Autodesk Fusion 360 part; units mm, degrees
note: some values were not read from the file. Chosen so that the rebuilt part matches the saved one: which bodies a step acts on.
(part 2 of 4)
  arc A344 (288.775, -83.4875) -> (288.275, -83.9875) centre (288.775, -83.9875) ccw
  arc A345 (302.275, -83.9875) -> (301.775, -83.4875) centre (301.775, -83.9875) ccw
  arc A346 (288.275, -96.9875) -> (288.775, -97.4875) centre (288.775, -96.9875) ccw
  arc A347 (301.775, -97.4875) -> (302.275, -96.9875) centre (301.775, -96.9875) ccw
  line L378 (5.4062, -102.5375) -> (18.4063, -102.5375)
  line L379 (5.4062, -116.5375) -> (18.4063, -116.5375)
  line L380 (4.9062, -103.0375) -> (4.9062, -116.0375)
  line L381 (18.9062, -103.0375) -> (18.9062, -116.0375)
  arc A348 (5.4062, -102.5375) -> (4.9062, -103.0375) centre (5.4062, -103.0375) ccw
  arc A349 (18.9062, -103.0375) -> (18.4062, -102.5375) centre (18.4062, -103.0375) ccw
  arc A350 (4.9062, -116.0375) -> (5.4062, -116.5375) centre (5.4062, -116.0375) ccw
  arc A351 (18.4062, -116.5375) -> (18.9063, -116.0375) centre (18.4062, -116.0375) ccw
  line L382 (29.2188, -102.5375) -> (42.2188, -102.5375)
  line L383 (29.2188, -116.5375) -> (42.2188, -116.5375)
  line L384 (28.7188, -103.0375) -> (28.7188, -116.0375)
  line L385 (42.7188, -103.0375) -> (42.7188, -116.0375)
  arc A352 (29.2188, -102.5375) -> (28.7187, -103.0375) centre (29.2188, -103.0375) ccw
  arc A353 (42.7188, -103.0375) -> (42.2188, -102.5375) centre (42.2188, -103.0375) ccw
  arc A354 (28.7188, -116.0375) -> (29.2188, -116.5375) centre (29.2188, -116.0375) ccw
  arc A355 (42.2188, -116.5375) -> (42.7188, -116.0375) centre (42.2188, -116.0375) ccw
  line L386 (55.4125, -102.5375) -> (68.4125, -102.5375)
  line L387 (55.4125, -116.5375) -> (68.4125, -116.5375)
  line L388 (54.9125, -103.0375) -> (54.9125, -116.0375)
  line L389 (68.9125, -103.0375) -> (68.9125, -116.0375)
  arc A356 (55.4125, -102.5375) -> (54.9125, -103.0375) centre (55.4125, -103.0375) ccw
  arc A357 (68.9125, -103.0375) -> (68.4125, -102.5375) centre (68.4125, -103.0375) ccw
  arc A358 (54.9125, -116.0375) -> (55.4125, -116.5375) centre (55.4125, -116.0375) ccw
  arc A359 (68.4125, -116.5375) -> (68.9125, -116.0375) centre (68.4125, -116.0375) ccw
  line L390 (129.2312, -102.5375) -> (142.2312, -102.5375)
  line L391 (129.2312, -116.5375) -> (142.2312, -116.5375)
  line L392 (128.7312, -103.0375) -> (128.7312, -116.0375)
  line L393 (142.7312, -103.0375) -> (142.7312, -116.0375)
  arc A360 (129.2312, -102.5375) -> (128.7312, -103.0375) centre (129.2312, -103.0375) ccw
  arc A361 (142.7312, -103.0375) -> (142.2312, -102.5375) centre (142.2312, -103.0375) ccw
  arc A362 (128.7312, -116.0375) -> (129.2312, -116.5375) centre (129.2312, -116.0375) ccw
  arc A363 (142.2312, -116.5375) -> (142.7312, -116.0375) centre (142.2312, -116.0375) ccw
  line L394 (82.9039, -103.8479) -> (88.5587, -103.8479)
  line L395 (89.0587, -104.3479) -> (89.0587, -106.7375)
  line L396 (89.5587, -107.2375) -> (135.7312, -107.2375)
  line L397 (135.7312, -111.8375) -> (89.5587, -111.8375)
  line L398 (89.0587, -112.3375) -> (89.0587, -115.6415)
  line L399 (88.5587, -116.1415) -> (87.7553, -116.1415)
  line L400 (87.2553, -116.6415) -> (87.2553, -116.8099)
  line L401 (86.7553, -117.3099) -> (84.7073, -117.3099)
  line L402 (84.2073, -116.8099) -> (84.2073, -116.6415)
  line L403 (83.7073, -116.1415) -> (82.9039, -116.1415)
  line L404 (82.4039, -115.6415) -> (82.4039, -110.5455)
  line L405 (81.9039, -110.0455) -> (81.5403, -110.0455)
  line L406 (81.5403, -110.0455) -> (81.5403, -107.7515)
  line L407 (82.0403, -107.2515) -> (82.4039, -107.2515)
  line L408 (82.4039, -107.2515) -> (82.4039, -104.3479)
  arc A364 (89.0587, -104.3479) -> (88.5587, -103.8479) centre (88.5587, -104.3479) ccw
  arc A365 (89.0587, -106.7375) -> (89.5587, -107.2375) centre (89.5587, -106.7375) ccw
  arc A366 (89.5587, -111.8375) -> (89.0587, -112.3375) centre (89.5587, -112.3375) ccw
  arc A367 (88.5587, -116.1415) -> (89.0587, -115.6415) centre (88.5587, -115.6415) ccw
  arc A368 (87.7553, -116.1415) -> (87.2553, -116.6415) centre (87.7553, -116.6415) ccw
  arc A369 (86.7553, -117.3099) -> (87.2552, -116.8099) centre (86.7553, -116.8099) ccw
  arc A370 (84.2073, -116.8099) -> (84.7073, -117.3099) centre (84.7073, -116.8099) ccw
  arc A371 (84.2073, -116.6415) -> (83.7073, -116.1415) centre (83.7073, -116.6415) ccw
  arc A372 (82.4039, -115.6415) -> (82.9039, -116.1415) centre (82.9039, -115.6415) ccw
  arc A373 (82.4039, -110.5455) -> (81.9039, -110.0455) centre (81.9039, -110.5455) ccw
  arc A374 (82.0403, -107.2515) -> (81.5402, -107.7515) centre (82.0403, -107.7515) ccw
  arc A375 (82.9039, -103.8479) -> (82.4039, -104.3479) centre (82.9039, -104.3479) ccw
  line L409 (188.5587, -103.8479) -> (182.9038, -103.8479)
  line L410 (182.4039, -104.3479) -> (182.4039, -106.7375)
  line L411 (181.9039, -107.2375) -> (135.7312, -107.2375)
  line L412 (135.7312, -111.8375) -> (181.9039, -111.8375)
  line L413 (182.4039, -112.3375) -> (182.4039, -115.6415)
  line L414 (182.9039, -116.1415) -> (183.7072, -116.1415)
  line L415 (184.2073, -116.6415) -> (184.2073, -116.8099)
  line L416 (184.7072, -117.3099) -> (186.7553, -117.3099)
  line L417 (187.2553, -116.8099) -> (187.2553, -116.6415)
  line L418 (187.7552, -116.1415) -> (188.5587, -116.1415)
  line L419 (189.0587, -115.6415) -> (189.0587, -110.5455)
  line L420 (189.5587, -110.0455) -> (189.9223, -110.0455)
  line L421 (189.9223, -110.0455) -> (189.9223, -107.7515)
  line L422 (189.4223, -107.2515) -> (189.0587, -107.2515)
  line L423 (189.0587, -107.2515) -> (189.0587, -104.3479)
  arc A376 (182.9039, -103.8479) -> (182.4039, -104.3479) centre (182.9039, -104.3479) ccw
  arc A377 (181.9039, -107.2375) -> (182.4039, -106.7375) centre (181.9039, -106.7375) ccw
  arc A378 (182.4039, -112.3375) -> (181.9039, -111.8375) centre (181.9039, -112.3375) ccw
  arc A379 (182.4039, -115.6415) -> (182.9039, -116.1415) centre (182.9039, -115.6415) ccw
  arc A380 (184.2072, -116.6415) -> (183.7072, -116.1415) centre (183.7072, -116.6415) ccw
  arc A381 (184.2073, -116.8099) -> (184.7072, -117.3099) centre (184.7072, -116.8099) ccw
  arc A382 (186.7552, -117.3099) -> (187.2552, -116.8099) centre (186.7552, -116.8099) ccw
  arc A383 (187.7552, -116.1415) -> (187.2552, -116.6415) centre (187.7552, -116.6415) ccw
  arc A384 (188.5587, -116.1415) -> (189.0587, -115.6415) centre (188.5587, -115.6415) ccw
  arc A385 (189.5587, -110.0455) -> (189.0587, -110.5455) centre (189.5587, -110.5455) ccw
  arc A386 (189.9223, -107.7515) -> (189.4223, -107.2515) centre (189.4223, -107.7515) ccw
  arc A387 (189.0587, -104.3479) -> (188.5587, -103.8479) centre (188.5587, -104.3479) ccw
  line L424 (203.05, -102.5375) -> (216.05, -102.5375)
  line L425 (203.05, -116.5375) -> (216.05, -116.5375)
  line L426 (202.55, -103.0375) -> (202.55, -116.0375)
  line L427 (216.55, -103.0375) -> (216.55, -116.0375)
  arc A388 (203.05, -102.5375) -> (202.55, -103.0375) centre (203.05, -103.0375) ccw
  arc A389 (216.55, -103.0375) -> (216.05, -102.5375) centre (216.05, -103.0375) ccw
  arc A390 (202.55, -116.0375) -> (203.05, -116.5375) centre (203.05, -116.0375) ccw
  arc A391 (216.05, -116.5375) -> (216.55, -116.0375) centre (216.05, -116.0375) ccw
  line L428 (229.2438, -102.5375) -> (242.2438, -102.5375)
  line L429 (229.2438, -116.5375) -> (242.2438, -116.5375)
  line L430 (228.7438, -103.0375) -> (228.7438, -116.0375)
  line L431 (242.7438, -103.0375) -> (242.7438, -116.0375)
  arc A392 (229.2438, -102.5375) -> (228.7438, -103.0375) centre (229.2438, -103.0375) ccw
  arc A393 (242.7438, -103.0375) -> (242.2438, -102.5375) centre (242.2438, -103.0375) ccw
  arc A394 (228.7438, -116.0375) -> (229.2438, -116.5375) centre (229.2438, -116.0375) ccw
  arc A395 (242.2438, -116.5375) -> (242.7438, -116.0375) centre (242.2438, -116.0375) ccw
  line L432 (250.675, -102.5375) -> (263.675, -102.5375)
  line L433 (250.675, -116.5375) -> (263.675, -116.5375)
  line L434 (250.175, -103.0375) -> (250.175, -116.0375)
  line L435 (264.175, -103.0375) -> (264.175, -116.0375)
  arc A396 (250.675, -102.5375) -> (250.175, -103.0375) centre (250.675, -103.0375) ccw
  arc A397 (264.175, -103.0375) -> (263.675, -102.5375) centre (263.675, -103.0375) ccw
  arc A398 (250.175, -116.0375) -> (250.675, -116.5375) centre (250.675, -116.0375) ccw
  arc A399 (263.675, -116.5375) -> (264.175, -116.0375) centre (263.675, -116.0375) ccw
  line L436 (269.725, -102.5375) -> (282.725, -102.5375)
  line L437 (269.725, -116.5375) -> (282.725, -116.5375)
  line L438 (269.225, -103.0375) -> (269.225, -116.0375)
  line L439 (283.225, -103.0375) -> (283.225, -116.0375)
  arc A400 (269.725, -102.5375) -> (269.225, -103.0375) centre (269.725, -103.0375) ccw
  arc A401 (283.225, -103.0375) -> (282.725, -102.5375) centre (282.725, -103.0375) ccw
  arc A402 (269.225, -116.0375) -> (269.725, -116.5375) centre (269.725, -116.0375) ccw
  arc A403 (282.725, -116.5375) -> (283.225, -116.0375) centre (282.725, -116.0375) ccw
  line L440 (288.775, -102.5375) -> (301.775, -102.5375)
  line L441 (288.775, -116.5375) -> (301.775, -116.5375)
  line L442 (288.275, -103.0375) -> (288.275, -116.0375)
  line L443 (302.275, -103.0375) -> (302.275, -116.0375)
  arc A404 (288.775, -102.5375) -> (288.275, -103.0375) centre (288.775, -103.0375) ccw
  arc A405 (302.275, -103.0375) -> (301.775, -102.5375) centre (301.775, -103.0375) ccw
  arc A406 (288.275, -116.0375) -> (288.775, -116.5375) centre (288.775, -116.0375) ccw
  arc A407 (301.775, -116.5375) -> (302.275, -116.0375) centre (301.775, -116.0375) ccw
  line L444 (0, -120.1996) -> (304.8, -120.1996)
  line L445 (0, 0) -> (304.8, 0)
  line L446 (0, -120.1996) -> (0, 0)
  line L447 (304.8, -120.1996) -> (304.8, 0)
  circle A408 centre (295.243, -9.275) radius 3.25
  line L448 (300.493, -15.275) -> (289.993, -15.275)
  line L449 (289.243, -14.525) -> (289.243, -4.025)
  line L450 (289.993, -3.275) -> (300.493, -3.275)
  line L451 (301.243, -4.025) -> (301.243, -14.525)
  line L452 (301.243, -15.275) -> (289.243, -3.275) construction
  line L453 (289.243, -15.275) -> (301.243, -3.275) construction
  arc A409 (301.243, -4.025) -> (300.493, -3.275) centre (300.493, -4.025) ccw
  arc A410 (300.493, -15.275) -> (301.243, -14.525) centre (300.493, -14.525) ccw
  arc A411 (289.243, -14.525) -> (289.993, -15.275) centre (289.993, -14.525) ccw
  arc A412 (289.993, -3.275) -> (289.243, -4.025) centre (289.993, -4.025) ccw
  line L454 (-4, 10) -> (308.8, 10)
  line L455 (308.8, 10) -> (308.8, -130.1996)
  line L456 (308.8, -130.1996) -> (-4, -130.1996)
  line L457 (-4, -130.1996) -> (-4, 10)
  line L458 (273.8, 10) -> (202.4, 10)
  line L459 (202.4, 10) -> (202.4, 3)
  line L460 (202.4, 3) -> (273.8, 3)
  line L461 (273.8, 3) -> (273.8, 10)
  line L462 (31, 10) -> (102.4, 10)
  line L463 (102.4, 10) -> (102.4, 3)
  line L464 (102.4, 3) -> (31, 3)
  line L465 (31, 3) -> (31, 10)
  line L466 (152.4, 0) -> (152.4, 19)
  line L467 (31, -130.1996) -> (102.4, -130.1996)
  line L468 (102.4, -130.1996) -> (102.4, -123.1996)
  line L469 (102.4, -123.1996) -> (31, -123.1996)
  line L470 (31, -123.1996) -> (31, -130.1996)
  line L471 (273.8, -130.1996) -> (202.4, -130.1996)
  line L472 (202.4, -130.1996) -> (202.4, -123.1996)
  line L473 (202.4, -123.1996) -> (273.8, -123.1996)
  line L474 (273.8, -123.1996) -> (273.8, -130.1996)
  line L475 (152.4, -120.1996) -> (152.4, -154.1242)
  point P0 (295.243, -9.275)
  dimension "d1" = 6.5
  dimension "d6" = 12
  dimension "d7" = 0.75
  dimension "d9" = 12
  dimension "d10" = 7
  dimension "d11" = 14
  dimension "d12" = 6.7539
  dimension "d13" = 10
  dimension "d14" = 4
  dimension "d15" = 10
  dimension "d16" = 4
  dimension "d19" = 2.525
  dimension "d20" = 2.525
  dimension "d21" = 35
  dimension "d22" = 7
  dimension "d23" = 100
  dimension "d24" = 35
  dimension "d25" = 7
  dimension "d26" = 50
  dimension "d27" = 35
  dimension "d28" = 35
  dimension "d29" = 100
  dimension "d30" = 50
  dimension "d31" = 7
  dimension "d32" = 7
  dimension "d37" = 71.4
  constraint horizontal L448
  constraint perpendicular L448 L449
  constraint parallel L448 L450
  constraint parallel L449 L451
  constraint coincident L452 P0
  constraint coincident L453 P0
  constraint coincident P0 A408.centre
  constraint coincident L453.end L451
  constraint coincident L453.end L450
  constraint tangent L451 A409
  constraint tangent L450 A409
  constraint coincident L452.start L448
  constraint coincident L452.start L451
  constraint tangent L448 A410
  constraint tangent L451 A410
  constraint equal A409 A410
  constraint coincident L453.start L449
  constraint coincident L453.start L448
  constraint tangent L449 A411
  constraint tangent L448 A411
  constraint equal A409 A411
  constraint coincident L452.end L449
  constraint coincident L452.end L450
  constraint tangent L449 A412
  constraint tangent L450 A412
  constraint equal A409 A412
  constraint horizontal L454
  constraint vertical L455
  constraint horizontal L456
  constraint vertical L457
  constraint horizontal L458
  constraint vertical L459
  constraint horizontal L460
  constraint vertical L461
  constraint coincident L454 L458.start
  constraint horizontal L462
  constraint vertical L463
  constraint horizontal L464
  constraint vertical L465
  constraint coincident L454 L462.start
  constraint midpoint L445 L466.start
  constraint perpendicular L454 L466
  constraint horizontal L467
  constraint vertical L468
  constraint horizontal L469
  constraint vertical L470
  constraint coincident L456 L467.start
  constraint horizontal L471
  constraint vertical L472
  constraint horizontal L473
  constraint vertical L474
  constraint coincident L456 L471.start
  constraint equal L460 L473
  constraint equal L464 L469
  constraint midpoint L444 L475.start
  constraint perpendicular L456 L475
  measures "d1" diameter of A408
  measures "d6" distance of L453.start L452.end
  measures "d7" radius of A409
  measures "d9" distance of L451.start L449.end
  measures "d10" distance of L54 P0
  measures "d11" distance of L50 L51
  measures "d12" distance of L52 P0
  measures "d13" distance of L444 L456
  measures "d14" distance of L447 L455
  measures "d15" distance of L445 L454
  measures "d16" distance of L446 L457
  measures "d19" distance of L2 L446
  measures "d20" distance of L145 L447
  measures "d21" distance of L454.start L462.start
  measures "d22" distance of L454 L464
  measures "d23" distance of L459 L463
  measures "d24" distance of L455 L461
  measures "d25" distance of L454 L460
  measures "d26" distance of L463 L466
  measures "d27" distance of L455.end L471.start
  measures "d28" distance of L456.end L467.start
  measures "d29" distance of L467.end L471.end
  measures "d30" distance of L467.end L475
  measures "d31" distance of L467 L469
  measures "d32" distance of L471 L473
  measures "d37" distance of L463 L465
extrude "Extrude1" add sketch "Plate May 11 2026" along normal blind 3 contours L444 L445 L446 L447 | L444 L445 L446 L454 L456 L457 L463 L464 L465 L466 L468 L469 L470 L475 | L444 L445 L447 L454 L455 L456 L459 L460 L461 L466 L472 L473 L474 L475 makes body 1
fillet "Fillet1" radius 5 4 edges at (308.8, -130.1996, 1.5) (-4, -130.1996, 1.5) (308.8, 10, 1.5) (-4, 10, 1.5) on bodies 1
fillet "Fillet2" radius 5 4 edges at (31, 10, 1.5) (202.4, 10, 1.5) (102.4, 10, 1.5) (273.8, 10, 1.5) on bodies 1
fillet "Fillet3" radius 5 4 edges at (273.8, -130.1996, 1.5) (202.4, -130.1996, 1.5) (102.4, -130.1996, 1.5) (31, -130.1996, 1.5) on bodies 1
ref_plane "WorkPlane1" through (156.4, 0, 0) normal (1, 0, 0) x (0, 1, 0)
sketch "Sketch2" plane through (0, 0, 0) normal (0, 0, -1) x (1, 0, 0)
  arc A0 (216.8375, 83.9875) -> (217.3375, 83.4875) centre (217.3375, 83.9875) ccw
  line L0 (216.8375, 83.9875) -> (216.8375, 96.9875)
  arc A1 (217.3375, 97.4875) -> (216.8375, 96.9875) centre (217.3375, 96.9875) ccw
  line L1 (217.3375, 97.4875) -> (230.3375, 97.4875)
  arc A2 (230.8375, 96.9875) -> (230.3375, 97.4875) centre (230.3375, 96.9875) ccw
  line L2 (230.8375, 96.9875) -> (230.8375, 83.9875)
  arc A3 (230.3375, 83.4875) -> (230.8375, 83.9875) centre (230.3375, 83.9875) ccw
  line L3 (230.3375, 83.4875) -> (217.3375, 83.4875)
  arc A4 (50.15, 45.8875) -> (50.65, 45.3875) centre (50.65, 45.8875) ccw
  line L4 (50.15, 45.8875) -> (50.15, 58.8875)
  arc A5 (50.65, 59.3875) -> (50.15, 58.8875) centre (50.65, 58.8875) ccw
  line L5 (50.65, 59.3875) -> (63.65, 59.3875)
  arc A6 (64.15, 58.8875) -> (63.65, 59.3875) centre (63.65, 58.8875) ccw
  line L6 (64.15, 58.8875) -> (64.15, 45.8875)
  arc A7 (63.65, 45.3875) -> (64.15, 45.8875) centre (63.65, 45.8875) ccw
  line L7 (63.65, 45.3875) -> (50.65, 45.3875)
  arc A8 (288.275, 26.8375) -> (288.775, 26.3375) centre (288.775, 26.8375) ccw
  line L8 (288.275, 26.8375) -> (288.275, 39.8375)
  arc A9 (288.775, 40.3375) -> (288.275, 39.8375) centre (288.775, 39.8375) ccw
  line L9 (288.775, 40.3375) -> (301.775, 40.3375)
  arc A10 (302.275, 39.8375) -> (301.775, 40.3375) centre (301.775, 39.8375) ccw
  line L10 (302.275, 39.8375) -> (302.275, 26.8375)
  arc A11 (301.775, 26.3375) -> (302.275, 26.8375) centre (301.775, 26.8375) ccw
  line L11 (301.775, 26.3375) -> (288.775, 26.3375)
  arc A12 (169.2125, 64.9375) -> (169.7125, 64.4375) centre (169.7125, 64.9375) ccw
  line L12 (169.2125, 64.9375) -> (169.2125, 77.9375)
  arc A13 (169.7125, 78.4375) -> (169.2125, 77.9375) centre (169.7125, 77.9375) ccw
  line L13 (169.7125, 78.4375) -> (182.7125, 78.4375)
  arc A14 (183.2125, 77.9375) -> (182.7125, 78.4375) centre (182.7125, 77.9375) ccw
  line L14 (183.2125, 77.9375) -> (183.2125, 64.9375)
  arc A15 (182.7125, 64.4375) -> (183.2125, 64.9375) centre (182.7125, 64.9375) ccw
  line L15 (182.7125, 64.4375) -> (169.7125, 64.4375)
  arc A16 (31.1, 45.8875) -> (31.6, 45.3875) centre (31.6, 45.8875) ccw
  line L16 (31.1, 45.8875) -> (31.1, 58.8875)
  arc A17 (31.6, 59.3875) -> (31.1, 58.8875) centre (31.6, 58.8875) ccw
  line L17 (31.6, 59.3875) -> (44.6, 59.3875)
  arc A18 (45.1, 58.8875) -> (44.6, 59.3875) centre (44.6, 58.8875) ccw
  line L18 (45.1, 58.8875) -> (45.1, 45.8875)
  arc A19 (44.6, 45.3875) -> (45.1, 45.8875) centre (44.6, 45.8875) ccw
  line L19 (44.6, 45.3875) -> (31.6, 45.3875)
  arc A20 (7.2875, 45.8875) -> (7.7875, 45.3875) centre (7.7875, 45.8875) ccw
  line L20 (7.2875, 45.8875) -> (7.2875, 58.8875)
  arc A21 (7.7875, 59.3875) -> (7.2875, 58.8875) centre (7.7875, 58.8875) ccw
  line L21 (7.7875, 59.3875) -> (20.7875, 59.3875)
  arc A22 (21.2875, 58.8875) -> (20.7875, 59.3875) centre (20.7875, 58.8875) ccw
  line L22 (21.2875, 58.8875) -> (21.2875, 45.8875)
  arc A23 (20.7875, 45.3875) -> (21.2875, 45.8875) centre (20.7875, 45.8875) ccw
  line L23 (20.7875, 45.3875) -> (7.7875, 45.3875)
  arc A24 (54.9125, 103.0375) -> (55.4125, 102.5375) centre (55.4125, 103.0375) ccw
  line L24 (54.9125, 103.0375) -> (54.9125, 116.0375)
  arc A25 (55.4125, 116.5375) -> (54.9125, 116.0375) centre (55.4125, 116.0375) ccw
  line L25 (55.4125, 116.5375) -> (68.4125, 116.5375)
  arc A26 (68.9125, 116.0375) -> (68.4125, 116.5375) centre (68.4125, 116.0375) ccw
  line L26 (68.9125, 116.0375) -> (68.9125, 103.0375)
  arc A27 (68.4125, 102.5375) -> (68.9125, 103.0375) centre (68.4125, 103.0375) ccw
  line L27 (68.4125, 102.5375) -> (55.4125, 102.5375)
  arc A28 (54.9125, 3.025) -> (55.4125, 2.525) centre (55.4125, 3.025) ccw
  line L28 (54.9125, 3.025) -> (54.9125, 16.025)
  arc A29 (55.4125, 16.525) -> (54.9125, 16.025) centre (55.4125, 16.025) ccw
  line L29 (55.4125, 16.525) -> (68.4125, 16.525)
  arc A30 (68.9125, 16.025) -> (68.4125, 16.525) centre (68.4125, 16.025) ccw
  line L30 (68.9125, 16.025) -> (68.9125, 3.025)
  arc A31 (68.4125, 2.525) -> (68.9125, 3.025) centre (68.4125, 3.025) ccw
  line L31 (68.4125, 2.525) -> (55.4125, 2.525)
  arc A32 (288.275, 64.9375) -> (288.775, 64.4375) centre (288.775, 64.9375) ccw
  line L32 (288.275, 64.9375) -> (288.275, 77.9375)
  arc A33 (288.775, 78.4375) -> (288.275, 77.9375) centre (288.775, 77.9375) ccw
  line L33 (288.775, 78.4375) -> (301.775, 78.4375)
  arc A34 (302.275, 77.9375) -> (301.775, 78.4375) centre (301.775, 77.9375) ccw
  line L34 (302.275, 77.9375) -> (302.275, 64.9375)
  arc A35 (301.775, 64.4375) -> (302.275, 64.9375) centre (301.775, 64.9375) ccw
  line L35 (301.775, 64.4375) -> (288.775, 64.4375)
  arc A36 (269.225, 83.9875) -> (269.725, 83.4875) centre (269.725, 83.9875) ccw
  line L36 (269.225, 83.9875) -> (269.225, 96.9875)
  arc A37 (269.725, 97.4875) -> (269.225, 96.9875) centre (269.725, 96.9875) ccw
  line L37 (269.725, 97.4875) -> (282.725, 97.4875)
  arc A38 (283.225, 96.9875) -> (282.725, 97.4875) centre (282.725, 96.9875) ccw
  line L38 (283.225, 96.9875) -> (283.225, 83.9875)
  arc A39 (282.725, 83.4875) -> (283.225, 83.9875) centre (282.725, 83.9875) ccw
  line L39 (282.725, 83.4875) -> (269.725, 83.4875)
  arc A40 (73.9625, 3.025) -> (74.4625, 2.525) centre (74.4625, 3.025) ccw
  line L40 (73.9625, 3.025) -> (73.9625, 16.025)
  arc A41 (74.4625, 16.525) -> (73.9625, 16.025) centre (74.4625, 16.025) ccw
  line L41 (74.4625, 16.525) -> (87.4625, 16.525)
  arc A42 (87.9625, 16.025) -> (87.4625, 16.525) centre (87.4625, 16.025) ccw
  line L42 (87.9625, 16.025) -> (87.9625, 3.025)
  arc A43 (87.4625, 2.525) -> (87.9625, 3.025) centre (87.4625, 3.025) ccw
  line L43 (87.4625, 2.525) -> (74.4625, 2.525)
  arc A44 (121.5875, 3.025) -> (122.0875, 2.525) centre (122.0875, 3.025) ccw
  line L44 (121.5875, 3.025) -> (121.5875, 16.025)
  arc A45 (122.0875, 16.525) -> (121.5875, 16.025) centre (122.0875, 16.025) ccw
  line L45 (122.0875, 16.525) -> (135.0875, 16.525)
  arc A46 (135.5875, 16.025) -> (135.0875, 16.525) centre (135.0875, 16.025) ccw
  line L46 (135.5875, 16.025) -> (135.5875, 3.025)
  arc A47 (135.0875, 2.525) -> (135.5875, 3.025) centre (135.0875, 3.025) ccw
  line L47 (135.0875, 2.525) -> (122.0875, 2.525)
  arc A48 (45.3875, 83.9875) -> (45.8875, 83.4875) centre (45.8875, 83.9875) ccw
  line L48 (45.3875, 83.9875) -> (45.3875, 96.9875)
  arc A49 (45.8875, 97.4875) -> (45.3875, 96.9875) centre (45.8875, 96.9875) ccw
  line L49 (45.8875, 97.4875) -> (58.8875, 97.4875)
  arc A50 (59.3875, 96.9875) -> (58.8875, 97.4875) centre (58.8875, 96.9875) ccw
  line L50 (59.3875, 96.9875) -> (59.3875, 83.9875)
  arc A51 (58.8875, 83.4875) -> (59.3875, 83.9875) centre (58.8875, 83.9875) ccw
  line L51 (58.8875, 83.4875) -> (45.8875, 83.4875)
  arc A52 (154.925, 26.8375) -> (155.425, 26.3375) centre (155.425, 26.8375) ccw
  line L52 (154.925, 26.8375) -> (154.925, 39.8375)
  arc A53 (155.425, 40.3375) -> (154.925, 39.8375) centre (155.425, 39.8375) ccw
  line L53 (155.425, 40.3375) -> (168.425, 40.3375)
  arc A54 (168.925, 39.8375) -> (168.425, 40.3375) centre (168.425, 39.8375) ccw
  line L54 (168.925, 39.8375) -> (168.925, 26.8375)
  arc A55 (168.425, 26.3375) -> (168.925, 26.8375) centre (168.425, 26.8375) ccw
  line L55 (168.425, 26.3375) -> (155.425, 26.3375)
  arc A56 (35.8625, 64.9375) -> (36.3625, 64.4375) centre (36.3625, 64.9375) ccw
  line L56 (35.8625, 64.9375) -> (35.8625, 77.9375)
  arc A57 (36.3625, 78.4375) -> (35.8625, 77.9375) centre (36.3625, 77.9375) ccw
  line L57 (36.3625, 78.4375) -> (49.3625, 78.4375)
  arc A58 (49.8625, 77.9375) -> (49.3625, 78.4375) centre (49.3625, 77.9375) ccw
  line L58 (49.8625, 77.9375) -> (49.8625, 64.9375)
  arc A59 (49.3625, 64.4375) -> (49.8625, 64.9375) centre (49.3625, 64.9375) ccw
  line L59 (49.3625, 64.4375) -> (36.3625, 64.4375)
  arc A60 (264.4625, 45.8875) -> (264.9625, 45.3875) centre (264.9625, 45.8875) ccw
  line L60 (264.4625, 45.8875) -> (264.4625, 58.8875)
  arc A61 (264.9625, 59.3875) -> (264.4625, 58.8875) centre (264.9625, 58.8875) ccw
  line L61 (264.9625, 59.3875) -> (277.9625, 59.3875)
  arc A62 (278.4625, 58.8875) -> (277.9625, 59.3875) centre (277.9625, 58.8875) ccw
  line L62 (278.4625, 58.8875) -> (278.4625, 45.8875)
  arc A63 (277.9625, 45.3875) -> (278.4625, 45.8875) centre (277.9625, 45.8875) ccw
  line L63 (277.9625, 45.3875) -> (264.9625, 45.3875)
  arc A64 (288.275, 45.8875) -> (288.775, 45.3875) centre (288.775, 45.8875) ccw
  line L64 (288.275, 45.8875) -> (288.275, 58.8875)
  arc A65 (288.775, 59.3875) -> (288.275, 58.8875) centre (288.775, 58.8875) ccw
  line L65 (288.775, 59.3875) -> (301.775, 59.3875)
  arc A66 (302.275, 58.8875) -> (301.775, 59.3875) centre (301.775, 58.8875) ccw
  line L66 (302.275, 58.8875) -> (302.275, 45.8875)
  arc A67 (301.775, 45.3875) -> (302.275, 45.8875) centre (301.775, 45.8875) ccw
  line L67 (301.775, 45.3875) -> (288.775, 45.3875)
  arc A68 (226.3625, 64.9375) -> (226.8625, 64.4375) centre (226.8625, 64.9375) ccw
  line L68 (226.3625, 64.9375) -> (226.3625, 77.9375)
  arc A69 (226.8625, 78.4375) -> (226.3625, 77.9375) centre (226.8625, 77.9375) ccw
  line L69 (226.8625, 78.4375) -> (239.8625, 78.4375)
  arc A70 (240.3625, 77.9375) -> (239.8625, 78.4375) centre (239.8625, 77.9375) ccw
  line L70 (240.3625, 77.9375) -> (240.3625, 64.9375)
  arc A71 (239.8625, 64.4375) -> (240.3625, 64.9375) centre (239.8625, 64.9375) ccw
  line L71 (239.8625, 64.4375) -> (226.8625, 64.4375)
  arc A72 (221.6, 45.8875) -> (222.1, 45.3875) centre (222.1, 45.8875) ccw
  line L72 (221.6, 45.8875) -> (221.6, 58.8875)
  arc A73 (222.1, 59.3875) -> (221.6, 58.8875) centre (222.1, 58.8875) ccw
  line L73 (222.1, 59.3875) -> (235.1, 59.3875)
  arc A74 (235.6, 58.8875) -> (235.1, 59.3875) centre (235.1, 58.8875) ccw
  line L74 (235.6, 58.8875) -> (235.6, 45.8875)
  arc A75 (235.1, 45.3875) -> (235.6, 45.8875) centre (235.1, 45.8875) ccw
  line L75 (235.1, 45.3875) -> (222.1, 45.3875)
  arc A76 (107.3, 45.8875) -> (107.8, 45.3875) centre (107.8, 45.8875) ccw
  line L76 (107.3, 45.8875) -> (107.3, 58.8875)
  arc A77 (107.8, 59.3875) -> (107.3, 58.8875) centre (107.8, 58.8875) ccw
  line L77 (107.8, 59.3875) -> (120.8, 59.3875)
  arc A78 (121.3, 58.8875) -> (120.8, 59.3875) centre (120.8, 58.8875) ccw
  line L78 (121.3, 58.8875) -> (121.3, 45.8875)
  arc A79 (120.8, 45.3875) -> (121.3, 45.8875) centre (120.8, 45.8875) ccw
  line L79 (120.8, 45.3875) -> (107.8, 45.3875)
  arc A80 (145.4, 45.8875) -> (145.9, 45.3875) centre (145.9, 45.8875) ccw
  line L80 (145.4, 45.8875) -> (145.4, 58.8875)
  arc A81 (145.9, 59.3875) -> (145.4, 58.8875) centre (145.9, 58.8875) ccw
  line L81 (145.9, 59.3875) -> (158.9, 59.3875)
  arc A82 (159.4, 58.8875) -> (158.9, 59.3875) centre (158.9, 58.8875) ccw
  line L82 (159.4, 58.8875) -> (159.4, 45.8875)
  arc A83 (158.9, 45.3875) -> (159.4, 45.8875) centre (158.9, 45.8875) ccw
  line L83 (158.9, 45.3875) -> (145.9, 45.3875)
  arc A84 (4.9062, 103.0375) -> (5.4062, 102.5375) centre (5.4062, 103.0375) ccw
  line L84 (4.9062, 103.0375) -> (4.9062, 116.0375)
  arc A85 (5.4062, 116.5375) -> (4.9062, 116.0375) centre (5.4062, 116.0375) ccw
  line L85 (5.4062, 116.5375) -> (18.4063, 116.5375)
  arc A86 (18.9063, 116.0375) -> (18.4062, 116.5375) centre (18.4062, 116.0375) ccw
  line L86 (18.9063, 116.0375) -> (18.9062, 103.0375)
  arc A87 (18.4062, 102.5375) -> (18.9063, 103.0375) centre (18.4062, 103.0375) ccw
  line L87 (18.4062, 102.5375) -> (5.4062, 102.5375)
  arc A88 (250.175, 103.0375) -> (250.675, 102.5375) centre (250.675, 103.0375) ccw
  line L88 (250.175, 103.0375) -> (250.175, 116.0375)
  arc A89 (250.675, 116.5375) -> (250.175, 116.0375) centre (250.675, 116.0375) ccw
  line L89 (250.675, 116.5375) -> (263.675, 116.5375)
  arc A90 (264.175, 116.0375) -> (263.675, 116.5375) centre (263.675, 116.0375) ccw
  line L90 (264.175, 116.0375) -> (264.175, 103.0375)
  arc A91 (263.675, 102.5375) -> (264.175, 103.0375) centre (263.675, 103.0375) ccw
  line L91 (263.675, 102.5375) -> (250.675, 102.5375)
  arc A92 (28.7187, 103.0375) -> (29.2188, 102.5375) centre (29.2188, 103.0375) ccw
  line L92 (28.7187, 103.0375) -> (28.7188, 116.0375)
  arc A93 (29.2188, 116.5375) -> (28.7188, 116.0375) centre (29.2188, 116.0375) ccw
  line L93 (29.2188, 116.5375) -> (42.2188, 116.5375)
  arc A94 (42.7188, 116.0375) -> (42.2188, 116.5375) centre (42.2188, 116.0375) ccw
  line L94 (42.7188, 116.0375) -> (42.7188, 103.0375)
  arc A95 (42.2188, 102.5375) -> (42.7188, 103.0375) centre (42.2188, 103.0375) ccw
  line L95 (42.2188, 102.5375) -> (29.2188, 102.5375)
  arc A96 (228.7438, 103.0375) -> (229.2438, 102.5375) centre (229.2438, 103.0375) ccw
  line L96 (228.7438, 103.0375) -> (228.7438, 116.0375)
  arc A97 (229.2438, 116.5375) -> (228.7438, 116.0375) centre (229.2438, 116.0375) ccw
  line L97 (229.2438, 116.5375) -> (242.2438, 116.5375)
  arc A98 (242.7438, 116.0375) -> (242.2438, 116.5375) centre (242.2438, 116.0375) ccw
  line L98 (242.7438, 116.0375) -> (242.7438, 103.0375)
  arc A99 (242.2438, 102.5375) -> (242.7438, 103.0375) centre (242.2438, 103.0375) ccw
  line L99 (242.2438, 102.5375) -> (229.2438, 102.5375)
  arc A100 (202.55, 103.0375) -> (203.05, 102.5375) centre (203.05, 103.0375) ccw
  line L100 (202.55, 103.0375) -> (202.55, 116.0375)
  arc A101 (203.05, 116.5375) -> (202.55, 116.0375) centre (203.05, 116.0375) ccw
  line L101 (203.05, 116.5375) -> (216.05, 116.5375)
  arc A102 (216.55, 116.0375) -> (216.05, 116.5375) centre (216.05, 116.0375) ccw
  line L102 (216.55, 116.0375) -> (216.55, 103.0375)
  arc A103 (216.05, 102.5375) -> (216.55, 103.0375) centre (216.05, 103.0375) ccw
  line L103 (216.05, 102.5375) -> (203.05, 102.5375)
  arc A104 (178.7375, 3.025) -> (179.2375, 2.525) centre (179.2375, 3.025) ccw
  line L104 (178.7375, 3.025) -> (178.7375, 16.025)
  arc A105 (179.2375, 16.525) -> (178.7375, 16.025) centre (179.2375, 16.025) ccw
  line L105 (179.2375, 16.525) -> (192.2375, 16.525)
  arc A106 (192.7375, 16.025) -> (192.2375, 16.525) centre (192.2375, 16.025) ccw
  line L106 (192.7375, 16.025) -> (192.7375, 3.025)
  arc A107 (192.2375, 2.525) -> (192.7375, 3.025) centre (192.2375, 3.025) ccw
  line L107 (192.2375, 2.525) -> (179.2375, 2.525)
  arc A108 (159.6875, 83.9875) -> (160.1875, 83.4875) centre (160.1875, 83.9875) ccw
  line L108 (159.6875, 83.9875) -> (159.6875, 96.9875)
  arc A109 (160.1875, 97.4875) -> (159.6875, 96.9875) centre (160.1875, 96.9875) ccw
  line L109 (160.1875, 97.4875) -> (173.1875, 97.4875)
  arc A110 (173.6875, 96.9875) -> (173.1875, 97.4875) centre (173.1875, 96.9875) ccw
  line L110 (173.6875, 96.9875) -> (173.6875, 83.9875)
  arc A111 (173.1875, 83.4875) -> (173.6875, 83.9875) centre (173.1875, 83.9875) ccw
  line L111 (173.1875, 83.4875) -> (160.1875, 83.4875)
  arc A112 (188.2625, 64.9375) -> (188.7625, 64.4375) centre (188.7625, 64.9375) ccw
  line L112 (188.2625, 64.9375) -> (188.2625, 77.9375)
  arc A113 (188.7625, 78.4375) -> (188.2625, 77.9375) centre (188.7625, 77.9375) ccw
  line L113 (188.7625, 78.4375) -> (201.7625, 78.4375)
  arc A114 (202.2625, 77.9375) -> (201.7625, 78.4375) centre (201.7625, 77.9375) ccw
  line L114 (202.2625, 77.9375) -> (202.2625, 64.9375)
  arc A115 (201.7625, 64.4375) -> (202.2625, 64.9375) centre (201.7625, 64.9375) ccw
  line L115 (201.7625, 64.4375) -> (188.7625, 64.4375)
  arc A116 (102.5375, 83.9875) -> (103.0375, 83.4875) centre (103.0375, 83.9875) ccw
  line L116 (102.5375, 83.9875) -> (102.5375, 96.9875)
  arc A117 (103.0375, 97.4875) -> (102.5375, 96.9875) centre (103.0375, 96.9875) ccw
  line L117 (103.0375, 97.4875) -> (116.0375, 97.4875)
  arc A118 (116.5375, 96.9875) -> (116.0375, 97.4875) centre (116.0375, 96.9875) ccw
  line L118 (116.5375, 96.9875) -> (116.5375, 83.9875)
  arc A119 (116.0375, 83.4875) -> (116.5375, 83.9875) centre (116.0375, 83.9875) ccw
  line L119 (116.0375, 83.4875) -> (103.0375, 83.4875)
  arc A120 (207.3125, 64.9375) -> (207.8125, 64.4375) centre (207.8125, 64.9375) ccw
  line L120 (207.3125, 64.9375) -> (207.3125, 77.9375)
  arc A121 (207.8125, 78.4375) -> (207.3125, 77.9375) centre (207.8125, 77.9375) ccw
  line L121 (207.8125, 78.4375) -> (220.8125, 78.4375)
  arc A122 (221.3125, 77.9375) -> (220.8125, 78.4375) centre (220.8125, 77.9375) ccw
  line L122 (221.3125, 77.9375) -> (221.3125, 64.9375)
  arc A123 (220.8125, 64.4375) -> (221.3125, 64.9375) centre (220.8125, 64.9375) ccw
  line L123 (220.8125, 64.4375) -> (207.8125, 64.4375)
  arc A124 (78.725, 26.8375) -> (79.225, 26.3375) centre (79.225, 26.8375) ccw
  line L124 (78.725, 26.8375) -> (78.725, 39.8375)
  arc A125 (79.225, 40.3375) -> (78.725, 39.8375) centre (79.225, 39.8375) ccw
  line L125 (79.225, 40.3375) -> (92.225, 40.3375)
  arc A126 (92.725, 39.8375) -> (92.225, 40.3375) centre (92.225, 39.8375) ccw
  line L126 (92.725, 39.8375) -> (92.725, 26.8375)
  arc A127 (92.225, 26.3375) -> (92.725, 26.8375) centre (92.225, 26.8375) ccw
  line L127 (92.225, 26.3375) -> (79.225, 26.3375)
  arc A128 (69.2, 45.8875) -> (69.7, 45.3875) centre (69.7, 45.8875) ccw
  line L128 (69.2, 45.8875) -> (69.2, 58.8875)
  arc A129 (69.7, 59.3875) -> (69.2, 58.8875) centre (69.7, 58.8875) ccw
  line L129 (69.7, 59.3875) -> (82.7, 59.3875)
  arc A130 (83.2, 58.8875) -> (82.7, 59.3875) centre (82.7, 58.8875) ccw
  line L130 (83.2, 58.8875) -> (83.2, 45.8875)
  arc A131 (82.7, 45.3875) -> (83.2, 45.8875) centre (82.7, 45.8875) ccw
  line L131 (82.7, 45.3875) -> (69.7, 45.3875)
  arc A132 (21.575, 26.8375) -> (22.075, 26.3375) centre (22.075, 26.8375) ccw
  line L132 (21.575, 26.8375) -> (21.575, 39.8375)
  arc A133 (22.075, 40.3375) -> (21.575, 39.8375) centre (22.075, 39.8375) ccw
  line L133 (22.075, 40.3375) -> (35.075, 40.3375)
  arc A134 (35.575, 39.8375) -> (35.075, 40.3375) centre (35.075, 39.8375) ccw
  line L134 (35.575, 39.8375) -> (35.575, 26.8375)
  arc A135 (35.075, 26.3375) -> (35.575, 26.8375) centre (35.075, 26.8375) ccw
  line L135 (35.075, 26.3375) -> (22.075, 26.3375)
  arc A136 (2.525, 26.8375) -> (3.025, 26.3375) centre (3.025, 26.8375) ccw
  line L136 (2.525, 26.8375) -> (2.525, 39.8375)
  arc A137 (3.025, 40.3375) -> (2.525, 39.8375) centre (3.025, 39.8375) ccw
  line L137 (3.025, 40.3375) -> (16.025, 40.3375)
  arc A138 (16.525, 39.8375) -> (16.025, 40.3375) centre (16.025, 39.8375) ccw
  line L138 (16.525, 39.8375) -> (16.525, 26.8375)
  arc A139 (16.025, 26.3375) -> (16.525, 26.8375) centre (16.025, 26.8375) ccw
  line L139 (16.025, 26.3375) -> (3.025, 26.3375)
  arc A140 (59.675, 26.8375) -> (60.175, 26.3375) centre (60.175, 26.8375) ccw
  line L140 (59.675, 26.8375) -> (59.675, 39.8375)
  arc A141 (60.175, 40.3375) -> (59.675, 39.8375) centre (60.175, 39.8375) ccw
  line L141 (60.175, 40.3375) -> (73.175, 40.3375)
  arc A142 (73.675, 39.8375) -> (73.175, 40.3375) centre (73.175, 39.8375) ccw
  line L142 (73.675, 39.8375) -> (73.675, 26.8375)
  arc A143 (73.175, 26.3375) -> (73.675, 26.8375) centre (73.175, 26.8375) ccw
  line L143 (73.175, 26.3375) -> (60.175, 26.3375)
  arc A144 (264.4625, 3.025) -> (264.9625, 2.525) centre (264.9625, 3.025) ccw
  line L144 (264.4625, 3.025) -> (264.4625, 16.025)
  arc A145 (264.9625, 16.525) -> (264.4625, 16.025) centre (264.9625, 16.025) ccw
  line L145 (264.9625, 16.525) -> (277.9625, 16.525)
  arc A146 (278.4625, 16.025) -> (277.9625, 16.525) centre (277.9625, 16.025) ccw
  line L146 (278.4625, 16.025) -> (278.4625, 3.025)
  arc A147 (277.9625, 2.525) -> (278.4625, 3.025) centre (277.9625, 3.025) ccw
  line L147 (277.9625, 2.525) -> (264.9625, 2.525)
  arc A148 (245.4125, 3.025) -> (245.9125, 2.525) centre (245.9125, 3.025) ccw
  line L148 (245.4125, 3.025) -> (245.4125, 16.025)
  arc A149 (245.9125, 16.525) -> (245.4125, 16.025) centre (245.9125, 16.025) ccw
  line L149 (245.9125, 16.525) -> (258.9125, 16.525)
  arc A150 (259.4125, 16.025) -> (258.9125, 16.525) centre (258.9125, 16.025) ccw
  line L150 (259.4125, 16.025) -> (259.4125, 3.025)
  arc A151 (258.9125, 2.525) -> (259.4125, 3.025) centre (258.9125, 3.025) ccw
  line L151 (258.9125, 2.525) -> (245.9125, 2.525)
  arc A152 (207.3125, 3.025) -> (207.8125, 2.525) centre (207.8125, 3.025) ccw
  line L152 (207.3125, 3.025) -> (207.3125, 16.025)
  arc A153 (207.8125, 16.525) -> (207.3125, 16.025) centre (207.8125, 16.025) ccw
  line L153 (207.8125, 16.525) -> (220.8125, 16.525)
  arc A154 (221.3125, 16.025) -> (220.8125, 16.525) centre (220.8125, 16.025) ccw
  line L154 (221.3125, 16.025) -> (221.3125, 3.025)
  arc A155 (220.8125, 2.525) -> (221.3125, 3.025) centre (220.8125, 3.025) ccw
  line L155 (220.8125, 2.525) -> (207.8125, 2.525)
  arc A156 (40.625, 26.8375) -> (41.125, 26.3375) centre (41.125, 26.8375) ccw
  line L156 (40.625, 26.8375) -> (40.625, 39.8375)
  arc A157 (41.125, 40.3375) -> (40.625, 39.8375) centre (41.125, 39.8375) ccw
  line L157 (41.125, 40.3375) -> (54.125, 40.3375)
  arc A158 (54.625, 39.8375) -> (54.125, 40.3375) centre (54.125, 39.8375) ccw
  line L158 (54.625, 39.8375) -> (54.625, 26.8375)
  arc A159 (54.125, 26.3375) -> (54.625, 26.8375) centre (54.125, 26.8375) ccw
  line L159 (54.125, 26.3375) -> (41.125, 26.3375)
  arc A160 (226.3625, 3.025) -> (226.8625, 2.525) centre (226.8625, 3.025) ccw
  line L160 (226.3625, 3.025) -> (226.3625, 16.025)
  arc A161 (226.8625, 16.525) -> (226.3625, 16.025) centre (226.8625, 16.025) ccw
  line L161 (226.8625, 16.525) -> (239.8625, 16.525)
  arc A162 (240.3625, 16.025) -> (239.8625, 16.525) centre (239.8625, 16.025) ccw
  line L162 (240.3625, 16.025) -> (240.3625, 3.025)
  arc A163 (239.8625, 2.525) -> (240.3625, 3.025) centre (239.8625, 3.025) ccw
  line L163 (239.8625, 2.525) -> (226.8625, 2.525)
  arc A164 (116.825, 26.8375) -> (117.325, 26.3375) centre (117.325, 26.8375) ccw
  line L164 (116.825, 26.8375) -> (116.825, 39.8375)
  arc A165 (117.325, 40.3375) -> (116.825, 39.8375) centre (117.325, 39.8375) ccw
  line L165 (117.325, 40.3375) -> (130.325, 40.3375)
  arc A166 (130.825, 39.8375) -> (130.325, 40.3375) centre (130.325, 39.8375) ccw
  line L166 (130.825, 39.8375) -> (130.825, 26.8375)
  arc A167 (130.325, 26.3375) -> (130.825, 26.8375) centre (130.325, 26.8375) ccw
  line L167 (130.325, 26.3375) -> (117.325, 26.3375)
  arc A168 (121.5875, 83.9875) -> (122.0875, 83.4875) centre (122.0875, 83.9875) ccw
  line L168 (121.5875, 83.9875) -> (121.5875, 96.9875)
  arc A169 (122.0875, 97.4875) -> (121.5875, 96.9875) centre (122.0875, 96.9875) ccw
  line L169 (122.0875, 97.4875) -> (135.0875, 97.4875)
  arc A170 (135.5875, 96.9875) -> (135.0875, 97.4875) centre (135.0875, 96.9875) ccw
  line L170 (135.5875, 96.9875) -> (135.5875, 83.9875)
  arc A171 (135.0875, 83.4875) -> (135.5875, 83.9875) centre (135.0875, 83.9875) ccw
  line L171 (135.0875, 83.4875) -> (122.0875, 83.4875)
  line L172 (189.5587, 110.0455) -> (189.9223, 110.0455)
  line L173 (189.9223, 110.0455) -> (189.9223, 107.7515)
  arc A172 (189.4223, 107.2515) -> (189.9223, 107.7515) centre (189.4223, 107.7515) ccw
  line L174 (189.4223, 107.2515) -> (189.0587, 107.2515)
  line L175 (189.0587, 107.2515) -> (189.0587, 104.3479)
  arc A173 (188.5587, 103.8479) -> (189.0587, 104.3479) centre (188.5587, 104.3479) ccw
  line L176 (188.5587, 103.8479) -> (182.9038, 103.8479)
  arc A174 (182.4039, 104.3479) -> (182.9039, 103.8479) centre (182.9039, 104.3479) ccw
  line L177 (182.4039, 104.3479) -> (182.4039, 106.7375)
  arc A175 (182.4039, 106.7375) -> (181.9039, 107.2375) centre (181.9039, 106.7375) ccw
  line L178 (181.9039, 107.2375) -> (142.7313, 107.2375)
  line L179 (142.7312, 107.2375) -> (142.7312, 103.0375)
  arc A176 (142.2312, 102.5375) -> (142.7312, 103.0375) centre (142.2312, 103.0375) ccw
  line L180 (142.2312, 102.5375) -> (129.2312, 102.5375)
  arc A177 (128.7312, 103.0375) -> (129.2312, 102.5375) centre (129.2312, 103.0375) ccw
  line L181 (128.7312, 103.0375) -> (128.7313, 107.2375)
  line L182 (128.7312, 107.2375) -> (89.5587, 107.2375)
  arc A178 (89.5587, 107.2375) -> (89.0587, 106.7375) centre (89.5587, 106.7375) ccw
  line L183 (89.0587, 106.7375) -> (89.0587, 104.3479)
  arc A179 (88.5587, 103.8479) -> (89.0587, 104.3479) centre (88.5587, 104.3479) ccw
  line L184 (88.5587, 103.8479) -> (82.9039, 103.8479)
  arc A180 (82.4039, 104.3479) -> (82.9039, 103.8479) centre (82.9039, 104.3479) ccw
  line L185 (82.4039, 104.3479) -> (82.4039, 107.2515)
  line L186 (82.4039, 107.2515) -> (82.0403, 107.2515)
  arc A181 (81.5402, 107.7515) -> (82.0403, 107.2515) centre (82.0403, 107.7515) ccw
  line L187 (81.5402, 107.7515) -> (81.5403, 110.0455)
  line L188 (81.5403, 110.0455) -> (81.9039, 110.0455)
  arc A182 (81.9039, 110.0455) -> (82.4039, 110.5455) centre (81.9038, 110.5455) ccw
  line L189 (82.4039, 110.5455) -> (82.4039, 115.6415)
  arc A183 (82.9039, 116.1415) -> (82.4039, 115.6415) centre (82.9039, 115.6415) ccw
  line L190 (82.9039, 116.1415) -> (83.7073, 116.1415)
  arc A184 (83.7073, 116.1415) -> (84.2073, 116.6415) centre (83.7073, 116.6415) ccw
  line L191 (84.2073, 116.6415) -> (84.2073, 116.8099)
  arc A185 (84.7073, 117.3099) -> (84.2073, 116.8099) centre (84.7073, 116.8099) ccw
  line L192 (84.7073, 117.3099) -> (86.7553, 117.3099)
  arc A186 (87.2552, 116.8099) -> (86.7553, 117.3099) centre (86.7553, 116.8099) ccw
  line L193 (87.2552, 116.8099) -> (87.2553, 116.6415)
  arc A187 (87.2553, 116.6415) -> (87.7553, 116.1415) centre (87.7552, 116.6415) ccw
  line L194 (87.7553, 116.1415) -> (88.5587, 116.1415)
  arc A188 (89.0587, 115.6415) -> (88.5587, 116.1415) centre (88.5587, 115.6415) ccw
  line L195 (89.0587, 115.6415) -> (89.0587, 112.3375)
  arc A189 (89.0587, 112.3375) -> (89.5587, 111.8375) centre (89.5587, 112.3375) ccw
  line L196 (89.5587, 111.8375) -> (128.7312, 111.8375)
  line L197 (128.7312, 111.8375) -> (128.7312, 116.0375)
  arc A190 (129.2312, 116.5375) -> (128.7312, 116.0375) centre (129.2312, 116.0375) ccw
  line L198 (129.2312, 116.5375) -> (142.2312, 116.5375)
  arc A191 (142.7312, 116.0375) -> (142.2312, 116.5375) centre (142.2312, 116.0375) ccw
  line L199 (142.7312, 116.0375) -> (142.7312, 111.8375)
  line L200 (142.7312, 111.8375) -> (181.9039, 111.8375)
  arc A192 (181.9039, 111.8375) -> (182.4039, 112.3375) centre (181.9039, 112.3375) ccw
  line L201 (182.4039, 112.3375) -> (182.4039, 115.6415)
  arc A193 (182.9039, 116.1415) -> (182.4039, 115.6415) centre (182.9039, 115.6415) ccw
  line L202 (182.9039, 116.1415) -> (183.7072, 116.1415)
  arc A194 (183.7072, 116.1415) -> (184.2072, 116.6415) centre (183.7072, 116.6415) ccw
  line L203 (184.2072, 116.6415) -> (184.2073, 116.8099)
  arc A195 (184.7072, 117.3099) -> (184.2073, 116.8099) centre (184.7072, 116.8099) ccw
  line L204 (184.7072, 117.3099) -> (186.7553, 117.3099)
  arc A196 (187.2552, 116.8099) -> (186.7552, 117.3099) centre (186.7552, 116.8099) ccw
  line L205 (187.2552, 116.8099) -> (187.2552, 116.6415)
  arc A197 (187.2552, 116.6415) -> (187.7552, 116.1415) centre (187.7552, 116.6415) ccw
  line L206 (187.7552, 116.1415) -> (188.5587, 116.1415)
  arc A198 (189.0587, 115.6415) -> (188.5587, 116.1415) centre (188.5587, 115.6415) ccw
  line L207 (189.0587, 115.6415) -> (189.0587, 110.5455)
  arc A199 (189.0587, 110.5455) -> (189.5587, 110.0455) centre (189.5587, 110.5455) ccw
  arc A200 (31, 125.1996) -> (26, 130.1996) centre (26, 125.1996) ccw
  line L208 (26, 130.1996) -> (1, 130.1996)
  arc A201 (1, 130.1996) -> (-4, 125.1996) centre (1, 125.1996) ccw
  line L209 (-4, 125.1996) -> (-4, -5)
  arc A202 (-4, -5) -> (1, -10) centre (1, -5) ccw
  line L210 (1, -10) -> (26, -10)
  arc A203 (26, -10) -> (31, -5) centre (26, -5) ccw
  line L211 (31, -5) -> (31, -3)
  line L212 (31, -3) -> (102.4, -3)
  line L213 (102.4, -3) -> (102.4, -5)
  arc A204 (102.4, -5) -> (107.4, -10) centre (107.4, -5) ccw
  line L214 (107.4, -10) -> (197.4, -10)
  arc A205 (197.4, -10) -> (202.4, -5) centre (197.4, -5) ccw
  line L215 (202.4, -5) -> (202.4, -3)
  line L216 (202.4, -3) -> (273.8, -3)
  line L217 (273.8, -3) -> (273.8, -5)
  arc A206 (273.8, -5) -> (278.8, -10) centre (278.8, -5) ccw
  line L218 (278.8, -10) -> (303.8, -10)
  arc A207 (303.8, -10) -> (308.8, -5) centre (303.8, -5) ccw
  line L219 (308.8, -5) -> (308.8, 125.1996)
  arc A208 (308.8, 125.1996) -> (303.8, 130.1996) centre (303.8, 125.1996) ccw
  line L220 (303.8, 130.1996) -> (278.8, 130.1996)
  arc A209 (278.8, 130.1996) -> (273.8, 125.1996) centre (278.8, 125.1996) ccw
  line L221 (273.8, 125.1996) -> (273.8, 123.1996)
  line L222 (273.8, 123.1996) -> (202.4, 123.1996)
  line L223 (202.4, 123.1996) -> (202.4, 125.1996)
  arc A210 (202.4, 125.1996) -> (197.4, 130.1996) centre (197.4, 125.1996) ccw
  line L224 (197.4, 130.1996) -> (107.4, 130.1996)
  arc A211 (107.4, 130.1996) -> (102.4, 125.1996) centre (107.4, 125.1996) ccw
  line L225 (102.4, 125.1996) -> (102.4, 123.1996)
  line L226 (102.4, 123.1996) -> (31, 123.1996)
  line L227 (31, 123.1996) -> (31, 125.1996)
  arc A212 (243.0313, 83.9875) -> (243.5313, 83.4875) centre (243.5313, 83.9875) ccw
  line L228 (243.0312, 83.9875) -> (243.0312, 96.9875)
  arc A213 (243.5313, 97.4875) -> (243.0313, 96.9875) centre (243.5313, 96.9875) ccw
  line L229 (243.5313, 97.4875) -> (256.5313, 97.4875)
  arc A214 (257.0312, 96.9875) -> (256.5312, 97.4875) centre (256.5312, 96.9875) ccw
  line L230 (257.0313, 96.9875) -> (257.0312, 83.9875)
  arc A215 (256.5312, 83.4875) -> (257.0312, 83.9875) centre (256.5312, 83.9875) ccw
  line L231 (256.5312, 83.4875) -> (243.5312, 83.4875)
  arc A216 (288.239, 3.025) -> (288.775, 2.5211) centre (288.7579, 3.04) ccw
  line L232 (288.239, 3.025) -> (288.2473, 16.025)
  arc A217 (288.775, 16.5282) -> (288.2473, 16.025) centre (288.7619, 16.0136) ccw
  line L233 (288.775, 16.5282) -> (301.775, 16.5283)
  arc A218 (302.2758, 16.025) -> (301.775, 16.5283) centre (301.7745, 16.0271) ccw
  line L234 (302.2758, 16.025) -> (302.2755, 3.025)
  arc A219 (301.775, 2.521) -> (302.2755, 3.025) centre (301.7743, 3.0222) ccw
  line L235 (301.775, 2.521) -> (288.775, 2.5211)
  arc A220 (135.875, 26.8375) -> (136.375, 26.3375) centre (136.375, 26.8375) ccw
  line L236 (135.875, 26.8375) -> (135.875, 39.8375)
  arc A221 (136.375, 40.3375) -> (135.875, 39.8375) centre (136.375, 39.8375) ccw
  line L237 (136.375, 40.3375) -> (149.375, 40.3375)
  arc A222 (149.875, 39.8375) -> (149.375, 40.3375) centre (149.375, 39.8375) ccw
  line L238 (149.875, 39.8375) -> (149.875, 26.8375)
  arc A223 (149.375, 26.3375) -> (149.875, 26.8375) centre (149.375, 26.8375) ccw
  line L239 (149.375, 26.3375) -> (136.375, 26.3375)
  arc A224 (73.9625, 64.9375) -> (74.4625, 64.4375) centre (74.4625, 64.9375) ccw
  line L240 (73.9625, 64.9375) -> (73.9625, 77.9375)
  arc A225 (74.4625, 78.4375) -> (73.9625, 77.9375) centre (74.4625, 77.9375) ccw
  line L241 (74.4625, 78.4375) -> (87.4625, 78.4375)
  arc A226 (87.9625, 77.9375) -> (87.4625, 78.4375) centre (87.4625, 77.9375) ccw
  line L242 (87.9625, 77.9375) -> (87.9625, 64.9375)
  arc A227 (87.4625, 64.4375) -> (87.9625, 64.9375) centre (87.4625, 64.9375) ccw
  line L243 (87.4625, 64.4375) -> (74.4625, 64.4375)
  arc A228 (126.35, 45.8875) -> (126.85, 45.3875) centre (126.85, 45.8875) ccw
  line L244 (126.35, 45.8875) -> (126.35, 58.8875)
  arc A229 (126.85, 59.3875) -> (126.35, 58.8875) centre (126.85, 58.8875) ccw
  line L245 (126.85, 59.3875) -> (139.85, 59.3875)
  arc A230 (140.35, 58.8875) -> (139.85, 59.3875) centre (139.85, 58.8875) ccw
  line L246 (140.35, 58.8875) -> (140.35, 45.8875)
  arc A231 (139.85, 45.3875) -> (140.35, 45.8875) centre (139.85, 45.8875) ccw
  line L247 (139.85, 45.3875) -> (126.85, 45.3875)
  line L248 (282.4654, 33.8455) -> (282.829, 33.8455)
  line L249 (282.829, 33.8455) -> (282.829, 31.5515)
  arc A232 (282.329, 31.0515) -> (282.829, 31.5515) centre (282.329, 31.5515) ccw
  line L250 (282.329, 31.0515) -> (281.9654, 31.0515)
  line L251 (281.9654, 31.0515) -> (281.9654, 28.1479)
  arc A233 (281.4654, 27.6479) -> (281.9654, 28.1479) centre (281.4654, 28.1479) ccw
  line L252 (281.4654, 27.6479) -> (275.8106, 27.6479)
  arc A234 (275.3106, 28.1479) -> (275.8106, 27.6479) centre (275.8106, 28.1479) ccw
  line L253 (275.3106, 28.1479) -> (275.3106, 28.4607)
  line L254 (275.3106, 28.4607) -> (273.7, 28.4607)
  line L255 (273.7, 28.4607) -> (273.7, 26.8375)
  arc A235 (273.2, 26.3375) -> (273.7, 26.8375) centre (273.2, 26.8375) ccw
  line L256 (273.2, 26.3375) -> (260.2, 26.3375)
  arc A236 (259.7, 26.8375) -> (260.2, 26.3375) centre (260.2, 26.8375) ccw
  line L257 (259.7, 26.8375) -> (259.7, 28.4607)
  line L258 (259.7, 28.4607) -> (258.0894, 28.4607)
  line L259 (258.0894, 28.4607) -> (258.0894, 28.1479)
  arc A237 (257.5894, 27.6479) -> (258.0894, 28.1479) centre (257.5894, 28.1479) ccw
  line L260 (257.5894, 27.6479) -> (251.9346, 27.6479)
  arc A238 (251.4346, 28.1479) -> (251.9346, 27.6479) centre (251.9346, 28.1479) ccw
  line L261 (251.4346, 28.1479) -> (251.4346, 31.0515)
  line L262 (251.4346, 31.0515) -> (251.071, 31.0515)
  arc A239 (250.571, 31.5515) -> (251.071, 31.0515) centre (251.071, 31.5515) ccw
  line L263 (250.571, 31.5515) -> (250.571, 33.8455)
  line L264 (250.571, 33.8455) -> (250.9346, 33.8455)
  arc A240 (250.9346, 33.8455) -> (251.4346, 34.3455) centre (250.9346, 34.3455) ccw
  line L265 (251.4346, 34.3455) -> (251.4346, 39.4415)
  arc A241 (251.9346, 39.9415) -> (251.4346, 39.4415) centre (251.9346, 39.4415) ccw
  line L266 (251.9346, 39.9415) -> (252.738, 39.9415)
  arc A242 (252.738, 39.9415) -> (253.238, 40.4415) centre (252.738, 40.4415) ccw
  line L267 (253.238, 40.4415) -> (253.238, 40.6099)
  arc A243 (253.738, 41.1099) -> (253.238, 40.6099) centre (253.738, 40.6099) ccw
  line L268 (253.738, 41.1099) -> (255.786, 41.1099)
  arc A244 (256.286, 40.6099) -> (255.786, 41.1099) centre (255.786, 40.6099) ccw
  line L269 (256.286, 40.6099) -> (256.286, 40.4415)
  arc A245 (256.286, 40.4415) -> (256.786, 39.9415) centre (256.786, 40.4415) ccw
  line L270 (256.786, 39.9415) -> (258.0894, 39.9415)
  line L271 (258.0894, 39.9415) -> (258.0894, 39.6541)
  arc A246 (258.0894, 39.6541) -> (258.5894, 39.1541) centre (258.5894, 39.6541) ccw
  line L272 (258.5894, 39.1541) -> (259.7, 39.1541)
  line L273 (259.7, 39.1541) -> (259.7, 39.8375)